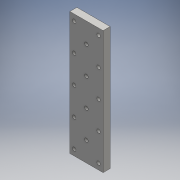
# Autodesk Inventor part: BearingSilicone_Base
Saved by Autodesk Inventor 2016 (Build 200138000, 138)
## iProperties
Created: 2015-12-22
Part Number: BearingSilicone_Base
Material: Generic
Document SubType Name: Modeling
Designer: momem
Density: 1 g/cm^3
Appearance: Default
Author: momem
Autodesk Inventor part; units mm, degrees
ref_plane "YZ Plane" through (0, 0, 0) normal (1, 0, 0) x (0, 1, 0)
ref_plane "XZ Plane" through (0, 0, 0) normal (0, 1, 0) x (-1, 0, 0)
ref_plane "XY Plane" through (0, 0, 0) normal (0, 0, 1) x (1, 0, 0)
sketch "Sketch1" plane through (0, 0, 0) normal (0, 1, 0) x (-1, 0, 0)
  circle A0 centre (0, 0) radius 10.45 construction
  circle A1 centre (0, 0) radius 1.5875
  circle A2 centre (0, -25) radius 9.9 construction
  circle A3 centre (0, -25) radius 1.5875
  circle A4 centre (0, -50) radius 9.57 construction
  circle A5 centre (0, -50) radius 1.5875
  circle A6 centre (0, -75) radius 9.35 construction
  circle A7 centre (0, -75) radius 1.5875
  line L0 (15, 18) -> (-15, 18)
  line L1 (-15, 18) -> (-15, -93)
  line L2 (-15, -93) -> (15, -93)
  line L3 (15, -93) -> (15, 18)
  circle A8 centre (0, 0) radius 11.45 construction
  circle A9 centre (0, -25) radius 10.9 construction
  circle A10 centre (0, -50) radius 10.57 construction
  circle A11 centre (0, -75) radius 10.35 construction
  circle A12 centre (11, -12.5) radius 1.5875
  line L4 (0, 0) -> (0, -25) construction
  line L5 (0, 0) -> (-15, 0) construction
  line L6 (0, -25) -> (-15, -25) construction
  line L7 (0, -50) -> (-15, -50) construction
  line L8 (0, -75) -> (-15, -75) construction
  circle A13 centre (-11, -12.5) radius 1.5875
  circle A14 centre (11, 12.5) radius 1.5875
  circle A15 centre (-11, 12.5) radius 1.5875
  circle A16 centre (11, -37.5) radius 1.5875
  circle A17 centre (-11, -37.5) radius 1.5875
  circle A18 centre (11, -62.5) radius 1.5875
  circle A19 centre (-11, -62.5) radius 1.5875
  circle A20 centre (11, -87.5) radius 1.5875
  circle A21 centre (-11, -87.5) radius 1.5875
  point P0 (0, -12.5)
  dimension "d0" = 20.9
  dimension "d1" = 3.175
  dimension "d2" = 19.8
  dimension "d3" = 3.175
  dimension "d4" = 19.14
  dimension "d5" = 3.175
  dimension "d6" = 18.7
  dimension "d7" = 3.175
  dimension "d8" = 25
  dimension "d9" = 25
  dimension "d10" = 25
  dimension "d11" = 15
  dimension "d12" = 15
  dimension "d13" = 18
  dimension "d14" = 18
  dimension "d15" = 1
  dimension "d16" = 1
  dimension "d17" = 1
  dimension "d18" = 1
  dimension "d19" = 3.175
  dimension "d20" = 4
  constraints: 22 centre point, 18 end point, 9 coincident, 9 symmetric about line, 4 perpendicular, 4 point on line, 3 parallel, 3 vertical alignment, 1 horizontal, 1 horizontal alignment, 1 midpoint, 1 vertical, 9 other
  measures "d0" diameter of A0
  measures "d1" diameter of A1
  measures "d2" diameter of A2
  measures "d3" diameter of A3
  measures "d4" diameter of A4
  measures "d5" diameter of A5
  measures "d6" diameter of A6
  measures "d7" diameter of A7
  measures "d8" distance of A3.centre point (0, 0)
  measures "d9" distance of A5.centre A3.centre
  measures "d10" distance of A7.centre A5.centre
  measures "d11" distance from line of A0.centre L3
  measures "d12" distance from line of L1 A0.centre
  measures "d13" distance from line of L2 A7.centre
  measures "d14" distance from line of point (0, 0) L0
  measures "d15" radial gap between concentric circles of A0 A8
  measures "d16" radial gap between concentric circles of A2 A9
  measures "d17" radial gap between concentric circles of A4 A10
  measures "d18" radial gap between concentric circles of A6 A11
  measures "d19" diameter of A12
  measures "d20" distance from line of L3 A12.centre
extrude "Extrusion2" add sketch "Sketch1" along normal blind 6.39
equation "\"d23\" = WoodThickness"
equation "\"WoodThickness\" = 6.39"
body "Solid2"
